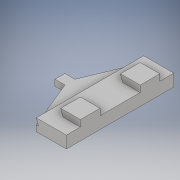
# Autodesk Inventor part: Tirador
Saved by Autodesk Inventor 2017 (Build 210142000, 142)
## iProperties
Created: 2017-01-19
Part Number: Tirador
Material: Generic
Document SubType Name: Modeling
Designer: A. Matías Quezada
Density: 1 g/cm^3
Appearance: Default
Author: A. Matías Quezada
Autodesk Inventor part; units mm, degrees
ref_plane "YZ Plane" through (0, 0, 0) normal (1, 0, 0) x (0, 1, 0)
ref_plane "XZ Plane" through (0, 0, 0) normal (0, 1, 0) x (-1, 0, 0)
ref_plane "XY Plane" through (0, 0, 0) normal (0, 0, 1) x (1, 0, 0)
sketch "Sketch1" plane through (0, 0, 0) normal (0, 0, 1) x (1, 0, 0)
  line L0 (0, 0) -> (-15, 0)
  line L1 (-15, 0) -> (-15, 53.6)
  line L2 (-15, 53.6) -> (0, 53.6)
  line L3 (0, 53.6) -> (0, 0)
  line L4 (-15, 53.6) -> (-25, 29.3)
  line L5 (-25, 29.3) -> (-30, 29.3)
  line L6 (-30, 29.3) -> (-30, 24.3)
  line L7 (-30, 24.3) -> (-25, 24.3)
  line L8 (-25, 24.3) -> (-15, 0)
  dimension "d0" = 15
  dimension "d1" = 53.6
  dimension "d2" = 5
  dimension "d15" = 10
  constraints: 18 end point, 3 equal length, 3 perpendicular, 2 horizontal, 2 parallel
  measures "d0" distance of L1.end L2.end
  measures "d1" distance of L0.end L1.end
  measures "d2" distance of L5.end L6.end
  measures "d15" horizontal distance of L7.end L0.end
extrude "Gancho" add sketch "Sketch1" along normal blind 3
sketch "Sketch2" plane through (0, 0, 3) normal (0, 0, 1) x (1, 0, 0)
  line L0 (-15, 0) -> (0, 0) projected
  line L1 (0, 0) -> (0, 53.6) projected
  line L2 (0, 53.6) -> (-15, 53.6) projected
  line L3 (-15, 53.6) -> (-15, 0)
  constraints: 2 end point, 1 vertical
extrude "Deslizador" add sketch "Sketch2" along normal blind 3
draft "Agarre Deslizador" angle -20 pull direction (0, 0, 1) faces at (-15, 17.8667, 4) fixed edges at (-15, 26.8, 6)
sketch "Sketch3" plane through (0, 0, 6) normal (0, 0, 1) x (1, 0, 0)
  line L0 (0, 53.6) -> (-15, 53.6) projected
  line L1 (-15, 0) -> (0, 0) projected
  line L2 (0, 0) -> (0, 53.6) projected
  line L3 (0, 0) -> (0, 53.6) projected
  line L4 (0, 7) -> (-9.8, 7)
  line L5 (-9.8, 7) -> (-9.8, 16.8)
  line L6 (-9.8, 16.8) -> (0, 16.8)
  line L7 (0, 36.8) -> (-9.8, 36.8)
  line L8 (-9.8, 36.8) -> (-9.8, 46.6)
  line L9 (-9.8, 46.6) -> (0, 46.6)
  line L10 (-9.8, 46.6) -> (-9.8, 53.6)
  line L11 (-9.8, 7) -> (-9.8, 0)
  point P0 (0, 43.8)
  point P1 (0, 9.8)
  dimension "d17" = 9.8
  dimension "d18" = 9.8
  dimension "d19" = 20
  constraints: 16 end point, 8 point on line, 7 perpendicular, 3 equal length, 1 vertical
  measures "d17" distance of L7.end L8.end
  measures "d18" distance of L8.end L9.end
  measures "d19" distance between parallel lines of L6 L7
extrude "Diente" add sketch "Sketch3" along normal blind 3.2 contours L2 L7 L8 L9 | L5 L6 L2 L4
draft "FaceDraft4" angle -20 pull direction (0, 0, 1) faces at (-9.8, 43.3333, 7.0667) fixed edges at (-9.8, 41.7, 9.2)
draft "FaceDraft5" angle -20 pull direction (0, 0, 1) faces at (-9.8, 13.5333, 8.1333) fixed edges at (-9.8, 11.9, 9.2)
equation "\"d0\" = tirador_deslizador_largo"
equation "\"d1\" = tirador_ancho"
equation "\"d2\" = tirador_gancho_ancho"
equation "\"d15\" = tirador_gancho_largo"
equation "\"d4\" = tirador_gancho_grosor"
equation "\"d6\" = tirador_deslizador_grosor"
equation "\"d8\" = tirador_deslizador_agarre"
equation "\"d17\" = tirador_diente_largo"
equation "\"d18\" = tirador_diente_largo"
equation "\"d20\" = tirador_diente_grosor"
equation "\"d22\" = tirador_diente_agarre"
equation "\"d23\" = tirador_diente_agarre"
equation "\"tirador_deslizador_largo\" = 15"
equation "\"tirador_ancho\" = 53.6"
equation "\"tirador_gancho_ancho\" = 5"
equation "\"tirador_gancho_largo\" = 10"
equation "\"tirador_gancho_grosor\" = 3"
equation "\"tirador_deslizador_grosor\" = 3"
equation "\"tirador_deslizador_agarre\" = -20deg"
equation "\"tirador_diente_largo\" = 9.8"
equation "\"tirador_diente_grosor\" = 3.2"
equation "\"tirador_diente_agarre\" = -20deg"
body "Solid1"
